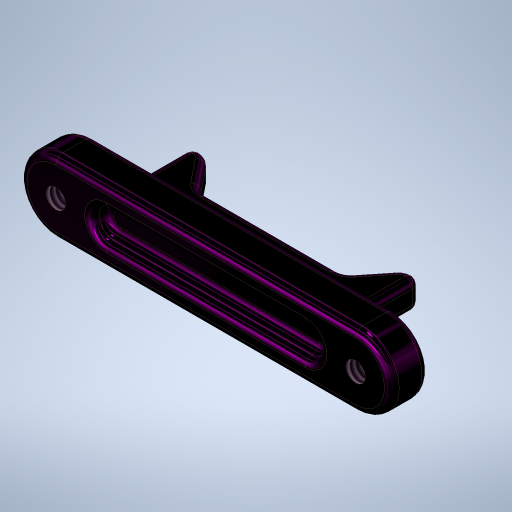
# Autodesk Inventor part: Front Shock Brace
Saved by Autodesk Inventor 2023.1 (Build 271208000, 208)
## iProperties
Created: 2019-11-26
Part Number: Front Shock Brace
Material: Generic
Document SubType Name: Modeling
Designer: Jopa
Density: 1 g/cm^3
Appearance: Brindle
Author: Jopa
Autodesk Inventor part; units mm, degrees
ref_plane "YZ Plane" through (0, 0, 0) normal (1, 0, 0) x (0, 1, 0)
ref_plane "XZ Plane" through (0, 0, 0) normal (0, 1, 0) x (-1, 0, 0)
sketch "Sketch1" plane through (0, 0, 0) normal (0, 0, 1) x (1, 0, 0)
  line L0 (0, -5.6007) -> (0, 5.6007) construction
  line L1 (-28.8036, 0) -> (28.8036, 0) construction
  line L2 (-16.5735, -4.0005) -> (16.5735, -4.0005)
  line L3 (16.5735, -4.0005) -> (16.5735, 4.0005) construction
  line L4 (16.5735, 4.0005) -> (-16.5735, 4.0005)
  line L5 (-16.5735, 4.0005) -> (-16.5735, -4.0005) construction
  line L6 (-16.5735, -4.0005) -> (16.5735, 4.0005) construction
  line L7 (16.5735, -4.0005) -> (-16.5735, 4.0005) construction
  arc A0 (16.5735, -4.0005) -> (16.5735, 4.0005) centre (16.5735, 0) ccw
  arc A1 (-16.5735, 4.0005) -> (-16.5735, -4.0005) centre (-16.5735, 0) ccw
  point P0 (0, 0)
  dimension "d1" = 8.001
  dimension "d2" = 33.147
  constraints: 12 end point, 4 point on circle, 4 tangent, 2 centre point, 2 midpoint, 2 parallel, 1 horizontal, 1 perpendicular
  measures "d1" distance of L4.end L2.start
  measures "d2" distance of L2.start L2.end
extrude "Extrusion1" add sketch "Sketch1" along normal blind 4.1275
sketch "Sketch2" plane through (0, 0, 4.1275) normal (0, 0, 1) x (1, 0, 0)
  line L0 (-10.9855, -1.5875) -> (10.9855, -1.5875)
  line L1 (10.9855, -1.5875) -> (10.9855, 1.5875) construction
  line L2 (10.9855, 1.5875) -> (-10.9855, 1.5875)
  line L3 (-10.9855, 1.5875) -> (-10.9855, -1.5875) construction
  line L4 (-10.9855, -1.5875) -> (10.9855, 1.5875) construction
  line L5 (10.9855, -1.5875) -> (-10.9855, 1.5875) construction
  arc A0 (-10.9855, 1.5875) -> (-10.9855, -1.5875) centre (-10.9855, 0) ccw
  arc A1 (10.9855, -1.5875) -> (10.9855, 1.5875) centre (10.9855, 0) ccw
  point P0 (0, 0)
  dimension "d5" = 21.971
  dimension "d6" = 3.175
  constraints: 12 end point, 4 point on circle, 4 tangent, 2 centre point, 2 midpoint, 2 parallel, 1 horizontal, 1 perpendicular
  measures "d5" distance of L0.start L0.end
  measures "d6" distance of L0.end L1.end
extrude "Extrusion2" cut sketch "Sketch2" against normal blind 1.5875
sketch "Sketch3" plane through (0, 0, 4.1275) normal (0, 0, 1) x (1, 0, 0)
  arc A0 (16.5735, -4.0005) -> (16.5735, 4.0005) centre (16.5735, 0) ccw projected
  arc A1 (-16.5735, 4.0005) -> (-16.5735, -4.0005) centre (-16.5735, 0) ccw projected
  point P0 (0, 0)
  constraints: 2 coincident
hole "Hole1" at (16.5735, 0, 4.1275) at (-16.5735, 0, 4.1275) direction (0, 0, -1) diameter 2.1565 end through all thread size "4-40 UNC" class "2B" standard "ANSI Unified Screw Threads"
ref_plane "Work Plane1" through (-16.5735, 0, -37.9939) normal (0, 1, 0) x (0, 0, 1)
sketch "Sketch4" plane through (-16.5735, 0, -37.9939) normal (0, 1, 0) x (0, 0, 1)
  line L0 (40.5339, 4.0005) -> (42.1214, 4.0005) projected
  line L1 (42.1214, 4.0005) -> (42.1214, 1.0782) projected
  line L2 (42.1214, 1.0782) -> (37.9939, 1.0782) projected
  line L3 (37.9939, 1.0782) -> (37.9939, 32.0688) projected
  line L4 (37.9939, 32.0688) -> (42.1214, 32.0688) projected
  line L5 (42.1214, 32.0688) -> (42.1214, 29.1465) projected
  line L6 (42.1214, 29.1465) -> (40.5339, 29.1465) projected
  line L7 (40.5339, 29.1465) -> (40.5339, 4.0005) projected
  line L8 (42.1214, -4.0005) -> (37.9939, -4.0005) projected
  line L9 (37.9939, -4.0005) -> (37.9939, -1.0782) projected
  line L10 (37.9939, -1.0782) -> (42.1214, -1.0782) projected
  line L11 (42.1214, -1.0782) -> (42.1214, -4.0005) projected
  line L12 (37.9939, 37.1475) -> (42.1214, 37.1475) projected
  line L13 (42.1214, 37.1475) -> (42.1214, 34.2252) projected
  line L14 (42.1214, 34.2252) -> (37.9939, 34.2252) projected
  line L15 (37.9939, 34.2252) -> (37.9939, 37.1475) projected
  line L16 (37.9939, 4.0005) -> (31.0089, 4.0005)
  line L17 (31.0089, 4.0005) -> (31.0089, 5.588)
  line L18 (31.0089, 5.588) -> (34.8189, 8.636)
  line L19 (34.8189, 8.636) -> (34.8189, 24.511)
  line L20 (28.7864, 16.5735) -> (44.3439, 16.5735) projected
  line L21 (37.9939, 29.1465) -> (31.0089, 29.1465)
  line L22 (31.0089, 29.1465) -> (31.0089, 27.559)
  line L23 (31.0089, 27.559) -> (34.8189, 24.511)
  line L24 (37.9939, 4.0005) -> (37.9939, 29.1465)
  line L25 (37.9939, 0) -> (37.9939, 33.147) projected
  point P0 (37.9939, 16.5735)
  point P1 (34.8189, 16.5735)
  point P2 (37.9939, 16.5735)
  dimension "d16" = 6.985
  dimension "d17" = 1.5875
  dimension "d18" = 15.875
  dimension "d19" = 3.175
  dimension "d20" = 8.001
  constraints: 16 end point, 3 symmetric about line, 2 midpoint, 1 collinear, 1 horizontal, 1 horizontal alignment, 1 parallel, 1 perpendicular, 1 point on line
  measures "d16" distance of L16.start L16.end
  measures "d17" distance of L16.end L17.end
  measures "d18" distance of L18.end L19.end
  measures "d19" distance between parallel lines of L3 L19
  measures "d20" distance between parallel lines of L16 L8
extrude "Extrusion3" add sketch "Sketch4" along normal mid plane 3.175 contours L20 L19 L23 L22 L21 L3 | L3 L16 L17 L18 L19 L20
fillet "Fillet1" radius 1.5875 4 edges at (-7.9375, 0, -3.175) (-10.9855, 0, -6.985) (10.9855, 0, -6.985) (7.9375, 0, -3.175)
fillet "Fillet2" radius 0.8128 4 edges at (12.573, 1.5875, -3.4925) (-12.573, 1.5875, -3.4925) (-12.573, -1.5875, -3.4925) (12.573, -1.5875, -3.4925)
fillet "Fillet3" radius 0.8128 48 edges at (-12.3349, 1.3494, 0) (-12.573, 0, 0) (-12.3349, -1.3494, 0) (0, -1.5875, 0) (12.3349, -1.3494, 0) (12.573, 0, 0) (12.3349, 1.3494, 0) (0, 1.5875, 0) (-7.8622, 1.5875, -3.3317) (-9.4615, 1.5875, -5.08) (-11.0608, 1.5875, -6.8283) (-11.7543, 1.5875, -6.985) (-12.3349, 1.3494, -6.985) (-12.573, 0, -6.985) (-12.3349, -1.3494, -6.985) (-11.7543, -1.5875, -6.985) (-11.0608, -1.5875, -6.8283) (-9.4615, -1.5875, -5.08) (-7.8622, -1.5875, -3.3317) (0, -1.5875, -3.175) (7.8622, -1.5875, -3.3317) (9.4615, -1.5875, -5.08) (11.0608, -1.5875, -6.8283) (11.7543, -1.5875, -6.985) (12.3349, -1.3494, -6.985) (12.573, 0, -6.985) (12.3349, 1.3494, -6.985) (11.7543, 1.5875, -6.985) (11.0608, 1.5875, -6.8283) (9.4615, 1.5875, -5.08) (7.8622, 1.5875, -3.3317) (0, 1.5875, -3.175) (-20.574, 0, 0) (0, -4.0005, 0) (20.574, 0, 0) (0, 4.0005, 0) (-20.574, 0, 4.1275) (0, -4.0005, 4.1275) (20.574, 0, 4.1275) (0, 4.0005, 4.1275) (-12.573, 0, 4.1275) (0, 1.5875, 4.1275) (12.573, 0, 4.1275) (0, -1.5875, 4.1275) (-12.573, 0, 2.54) (0, 1.5875, 2.54) (12.573, 0, 2.54) (0, -1.5875, 2.54)
body "Solid1"
